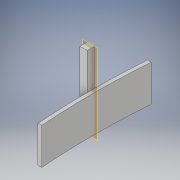
# Autodesk Inventor part: silothingp2
Saved by Autodesk Inventor 2019 (Build 230136000, 136)
## iProperties
Created: 2018-07-21
Part Number: silothingp2
Material: Generic
Document SubType Name: Modeling
Designer: Kitte_X
Density: 1 g/cm^3
Appearance: Default
Mass: 0.382458 g
Surface Area: 8.10621 cm^2
Volume: 0.382458 cm^3
Author: Kitte_X
Autodesk Inventor part; units mm, degrees
ref_plane "YZ Plane" through (0, 0, 0) normal (1, 0, 0) x (0, 1, 0)
ref_plane "XZ Plane" through (0, 0, 0) normal (0, 1, 0) x (-1, 0, 0)
ref_plane "XY Plane" through (0, 0, 0) normal (0, 0, 1) x (1, 0, 0)
sketch "Sketch1" plane through (0, 0, 0) normal (0, 1, 0) x (-1, 0, 0)
  arc A0 (0, -15) -> (0, 15) centre (-199.4367, 0) ccw
  line L0 (0, 15) -> (1, 15.0752)
  line L1 (0, -15) -> (1, -15.0752)
  arc A1 (1, -15.0752) -> (1, 15.0752) centre (-198.431, 0) ccw
  line L2 (1.5665, 1) -> (3.5665, 1)
  line L3 (3.5665, -1) -> (1.5665, -1)
  arc A2 (3.5665, -1) -> (3.5665, 1) centre (-196.431, 0) ccw
  point P0 (0, 0)
  point P1 (0.5633, 0)
  dimension "d0" = 200
  dimension "d1" = 30
  dimension "d2" = 1
  dimension "d3" = 1
  dimension "d4" = 200
  dimension "d5" = 1
  dimension "d6" = 1
  dimension "d7" = 2
  dimension "d8" = 2
  dimension "d9" = 200
  constraints: 9 point on circle, 8 end point, 3 centre point, 2 horizontal, 2 line through centre, 2 vertical alignment, 1 horizontal alignment
  measures "d0" radius of A0
  measures "d1" distance of L0.start L1.start
  measures "d2" horizontal distance of L0.start L0.end
  measures "d3" horizontal distance of L1.start L1.end
  measures "d4" radius of A1
  measures "d5" distance from line of point (0, 0) L2
  measures "d6" distance from line of L3 point (0, 0)
  measures "d7" distance of L2.start L2.end
  measures "d8" distance of L3.start L3.end
  measures "d9" radius of A2
extrude "Extrusion1" add sketch "Sketch1" along normal blind 20 contours A1 L2 A2 L3
extrude "Extrusion2" add sketch "Sketch1" along normal blind 10 contours A0 L0 A1 L1
ref_plane "Work Plane1" through (-3.5665, 20, 0) normal (0, 0, 1) x (1, 0, 0)
body "Solid1"
